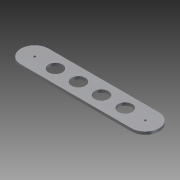
# Autodesk Inventor part: outer drive side
Saved by Autodesk Inventor 2011 (Build 150239000, 239)
## iProperties
Created: 2010-04-20
Part Number: outer drive side
Document SubType Name: Modeling
Designer: lucio
Density: 1 g/cm^3
Mass: 399 g
Surface Area: 977.264 cm^2
Volume: 399 cm^3
Author: lucio
Autodesk Inventor part; units mm, degrees
ref_plane "YZ Plane" through (0, 0, 0) normal (1, 0, 0) x (0, 1, 0)
ref_plane "XZ Plane" through (0, 0, 0) normal (0, 1, 0) x (-1, 0, 0)
ref_plane "XY Plane" through (0, 0, 0) normal (0, 0, 1) x (1, 0, 0)
sketch "Sketch1" plane through (0, 0, 0) normal (0, 0, 1) x (1, 0, 0)
  line L0 (-419.6966, 0.5698) -> (-19.6966, 0.5698)
  line L1 (-19.6966, 0.5698) -> (-19.6966, 100.5698)
  line L2 (-19.6966, 100.5698) -> (-419.6966, 100.5698)
  line L3 (-419.6966, 100.5698) -> (-419.6966, 0.5698)
  circle A0 centre (-419.6966, 50.5698) radius 50
  circle A1 centre (-19.6966, 50.5698) radius 50
  dimension "d12" = 400
  dimension "d13" = 100
  dimension "d14" = 100
  dimension "d15" = 100
  constraints: 8 end point, 2 centre point, 2 midpoint, 2 parallel, 1 horizontal, 1 perpendicular
  measures "d12" distance of L2.end L1.end
  measures "d13" distance of L1.end L0.end
  measures "d14" diameter of A0
  measures "d15" diameter of A1
extrude "Extrusion1" add sketch "Sketch1" along normal blind 10
sketch "Sketch2" plane through (0, 0, 10) normal (0, 0, 1) x (1, 0, 0)
  arc A0 (-419.6966, 100.5698) -> (-419.6966, 0.5698) centre (-419.6966, 50.5698) ccw projected
  arc A1 (-19.6966, 0.5698) -> (-19.6966, 100.5698) centre (-19.6966, 50.5698) ccw projected
  point P0 (0, 0)
  constraints: 2 coincident
hole "Hole1" at (-419.6966, 50.5698, 10) at (-19.6966, 50.5698, 10) direction (0, 0, -1) diameter 8 end through all
sketch "Sketch3" plane through (0, 0, 10) normal (0, 0, 1) x (1, 0, 0)
  circle A0 centre (-19.6966, 50.5698) radius 4 projected
  circle A1 centre (-419.6966, 50.5698) radius 4 projected
  line L0 (-19.6966, 0.5698) -> (-419.6966, 0.5698) projected
  circle A2 centre (-344.6966, 50.5698) radius 25
  circle A3 centre (-261.3633, 50.5698) radius 25
  circle A4 centre (-178.03, 50.5698) radius 25
  circle A5 centre (-94.6966, 52.8735) radius 25
  point P0 (0, 0)
  dimension "d16" = 50
  dimension "d17" = 50
  dimension "d18" = 50
  dimension "d19" = 50
  dimension "d20" = 83.3333
  dimension "d21" = 83.3333
  dimension "d22" = 83.3333
  dimension "d23" = 50
  dimension "d24" = 75
  dimension "d25" = 400
  constraints: 4 centre point
  measures "d16" diameter of A2
  measures "d17" diameter of A3
  measures "d18" diameter of A4
  measures "d19" diameter of A5
  measures "d20" distance of A3.centre A2.centre
  measures "d21" distance of A3.centre A4.centre
  measures "d22" horizontal distance of A5.centre A4.centre
  measures "d23" distance from line of L0 A2.centre
  measures "d24" distance of A1.centre A2.centre
  measures "d25" distance of A0.centre A1.centre
extrude "Extrusion2" cut sketch "Sketch3" against normal through all contours A2 | A3 | A4 | A5
equation "\"d14\" = d13"
equation "\"d15\" = d13"
equation "\"d17\" = d16"
equation "\"d18\" = d16"
equation "\"d19\" = d16"
equation "\"d20\" = -0.666667 * d24 + 0.333333 * d25"
equation "\"d21\" = d20"
equation "\"d22\" = d20"
body "Solid1"
